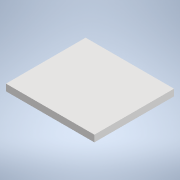
# Autodesk Inventor part: BodyClipMiddle
Saved by Autodesk Inventor 2020 (Build 240168000, 168)
## iProperties
Created: 2020-06-06
Part Number: BodyClipMiddle
Material: Generic
Document SubType Name: Modeling
Designer: user
Density: 1 g/cm^3
Appearance: Default
Author: user
Autodesk Inventor part; units mm, degrees
ref_plane "YZ Plane" through (0, 0, 0) normal (1, 0, 0) x (0, 1, 0)
ref_plane "XZ Plane" through (0, 0, 0) normal (0, 1, 0) x (-1, 0, 0)
ref_plane "XY Plane" through (0, 0, 0) normal (0, 0, 1) x (1, 0, 0)
sketch "Sketch1" plane through (0, 0, 0) normal (0, 1, 0) x (-1, 0, 0)
  line L0 (16.2488, 34.7042) -> (-17.0512, 34.7042)
  line L1 (-17.0512, 34.7042) -> (-17.0512, 4.7042)
  line L2 (-17.0512, 4.7042) -> (16.2488, 4.7042)
  line L3 (16.2488, 4.7042) -> (16.2488, 34.7042)
  point P0 (0, 0)
  dimension "d0" = 33.3
  dimension "d1" = 30
  constraints: 8 end point, 2 parallel, 1 horizontal, 1 perpendicular
  measures "d0" distance of L0.end L0.start
  measures "d1" distance of L2.end L0.start
extrude "Extrusion1" add sketch "Sketch1" along normal blind 2.5
equation "\"d2\" = ClipHeight"
equation "\"ClipHeight\" = 2.5"
body "Solid1"
